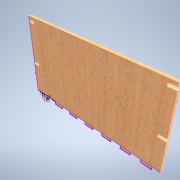
# Autodesk Inventor part: DoosjeVoorkant
Saved by Autodesk Inventor 2021 (Build 250183000, 183)
## iProperties
Created: 2021-03-11
Part Number: DoosjeVoorkant
Material: Wood (Cherry)
Document SubType Name: Modeling
Designer: ZiweZhang
Density: 0.63 g/cm^3
Appearance: Cherry - Natural Low Gloss
Author: ZiweZhang
Autodesk Inventor part; units mm, degrees
ref_plane "YZ Plane" through (0, 0, 0) normal (1, 0, 0) x (0, 1, 0)
ref_plane "XZ Plane" through (0, 0, 0) normal (0, 1, 0) x (-1, 0, 0)
ref_plane "XY Plane" through (0, 0, 0) normal (0, 0, 1) x (1, 0, 0)
sketch "Sketch1" plane through (0, 0, 0) normal (0, 0, 1) x (1, 0, 0)
  line L0 (0, 0) -> (144, 0)
  line L1 (144, 0) -> (144, 77)
  line L2 (144, 77) -> (0, 77)
  line L3 (0, 77) -> (0, 0)
  dimension "d0" = 144
  dimension "d1" = 77
  constraints: 8 end point, 2 parallel, 1 horizontal, 1 perpendicular
  measures "d0" distance of L2.end L1.end
  measures "d1" distance of L1.end L0.end
extrude "Extrusion1" add sketch "Sketch1" along normal blind 3
sketch "Sketch2" plane through (0, 0, 3) normal (0, 0, 1) x (1, 0, 0)
  line L0 (0, 0) -> (144, 0) projected
  line L1 (144, 0) -> (0, 0)
  line L2 (0, 0) -> (0, 77)
  line L3 (7, 0) -> (7, -3)
  line L4 (7, -3) -> (17, -3)
  line L5 (17, -3) -> (17, 0)
  line L6 (27, 0) -> (27, -3)
  line L7 (27, -3) -> (37, -3)
  line L8 (37, -3) -> (37, 0)
  line L9 (47, 0) -> (47, -3)
  line L10 (47, -3) -> (57, -3)
  line L11 (57, -3) -> (57, 0)
  line L12 (67, 0) -> (67, -3)
  line L13 (67, -3) -> (77, -3)
  line L14 (77, -3) -> (77, 0)
  line L15 (87, 0) -> (87, -3)
  line L16 (87, -3) -> (97, -3)
  line L17 (97, -3) -> (97, 0)
  line L18 (107, 0) -> (107, -3)
  line L19 (107, -3) -> (117, -3)
  line L20 (117, -3) -> (117, 0)
  line L21 (127, 0) -> (127, -3)
  line L22 (127, -3) -> (137, -3)
  line L23 (137, -3) -> (137, 0)
  line L24 (0, 77) -> (0, 0) projected
  point P0 (0, 20)
  dimension "d4" = 3
  dimension "d5" = 10
  dimension "d8" = 20
  constraints: 46 end point, 3 perpendicular, 3 point on line, 1 horizontal, 42 other
  measures "d4" distance of L3.start L3.end
  measures "d5" distance of L3.end L4.end
  measures "d8" distance of L3.start L6.start
extrude "Extrusion2" add sketch "Sketch2" against normal blind 3
sketch "Sketch3" plane through (0, 0, 3) normal (0, 0, 1) x (1, 0, 0)
  line L0 (0, 74) -> (7, 74)
  line L1 (7, 74) -> (7, 71)
  line L2 (7, 71) -> (0, 71)
  line L3 (0, 71) -> (0, 74)
  line L4 (137, 74) -> (144, 74)
  line L5 (144, 74) -> (144, 71)
  line L6 (144, 71) -> (137, 71)
  line L7 (137, 71) -> (137, 74)
  line L8 (0, 33) -> (7, 33)
  line L9 (7, 33) -> (7, 30)
  line L10 (7, 30) -> (0, 30)
  line L11 (0, 30) -> (0, 33)
  line L12 (137, 33) -> (144, 33)
  line L13 (144, 33) -> (144, 30)
  line L14 (144, 30) -> (137, 30)
  line L15 (137, 30) -> (137, 33)
  point P0 (0, 0)
  dimension "d27" = 7
  dimension "d28" = 3
  dimension "d31" = 137
  dimension "d34" = 41
  constraints: 32 end point, 3 perpendicular, 2 collinear, 2 horizontal, 1 vertical, 22 other
  measures "d27" distance of L0.start L0.end
  measures "d28" distance of L0.end L1.end
  measures "d31" distance of L0.start L4.start
  measures "d34" distance of L0.start L8.start
extrude "Extrusion3" cut sketch "Sketch3" against normal through all
body "Solid1"
